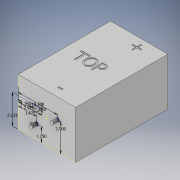
# Autodesk Inventor part: 12S Module
Saved by Autodesk Inventor 2017 (Build 210142000, 142)
## iProperties
Created: 2021-02-12
Part Number: 12S Module
Material: Generic
Document SubType Name: Modeling
Designer: Win240
Density: 1 g/cm^3
Appearance: Default
Author: Win240
Autodesk Inventor part; units mm, degrees
ref_plane "YZ Plane" through (0, 0, 0) normal (1, 0, 0) x (0, 1, 0)
ref_plane "XZ Plane" through (0, 0, 0) normal (0, 1, 0) x (-1, 0, 0)
ref_plane "XY Plane" through (0, 0, 0) normal (0, 0, 1) x (1, 0, 0)
sketch "Sketch1" plane through (0, 0, 0) normal (0, 0, 1) x (1, 0, 0)
  line L0 (-65.0875, -53.975) -> (65.0875, -53.975)
  line L1 (65.0875, -53.975) -> (65.0875, 53.975)
  line L2 (65.0875, 53.975) -> (-65.0875, 53.975)
  line L3 (-65.0875, 53.975) -> (-65.0875, -53.975)
  line L4 (-65.0875, -53.975) -> (65.0875, 53.975) construction
  line L5 (65.0875, -53.975) -> (-65.0875, 53.975) construction
  point P0 (0, 0)
  dimension "d0" = 130.175
  dimension "d1" = 107.95
  constraints: 12 end point, 2 midpoint, 2 parallel, 1 horizontal, 1 perpendicular
  measures "d0" distance of L0.start L0.end
  measures "d1" distance of L0.end L1.end
extrude "Extrusion1" add sketch "Sketch1" along normal blind 209.55
sketch "Sketch2" plane through (0, 0, 209.55) normal (0, 0, 1) x (1, 0, 0)
  line L0 (-65.0875, -53.975) -> (65.0875, -53.975) construction
  line L1 (-65.0875, 53.975) -> (-65.0875, -53.975) construction
  circle A0 centre (-23.8125, -22.225) radius 4
  circle A1 centre (23.8125, 9.525) radius 4
  line L2 (-11.1125, 12.065) -> (-33.3375, 12.065)
  line L3 (-33.3375, 12.065) -> (-33.3375, 13.335)
  line L4 (-33.3375, 13.335) -> (-11.1125, 13.335)
  line L5 (-11.1125, 13.335) -> (-11.1125, 12.065)
  line L6 (-33.3375, 12.7) -> (-65.0875, 12.7) construction
  point P0 (0, 0)
  dimension "d4" = 31.75
  dimension "d5" = 41.275
  dimension "d6" = 8
  dimension "d7" = 63.5
  dimension "d8" = 88.9
  dimension "d13" = 31.75
  dimension "d14" = 53.975
  dimension "d15" = 66.675
  dimension "d16" = 1.27
  constraints: 10 end point, 2 centre point, 2 horizontal, 2 parallel, 1 equal radius, 1 midpoint, 1 perpendicular, 1 point on line
  measures "d4" distance from line of A0.centre L0
  measures "d5" distance from line of A0.centre L1
  measures "d6" diameter of A0
  measures "d7" distance from line of A1.centre L0
  measures "d8" distance from line of A1.centre L1
  measures "d13" distance between parallel lines of L3 L1
  measures "d14" distance between parallel lines of L5 L1
  measures "d15" distance between parallel lines of L0 L6
  measures "d16" distance of L4.end L2.start
extrude "Extrusion2" add sketch "Sketch2" along normal blind 12.7
sketch "Sketch3" plane through (0, 0, 0) normal (0, 0, -1) x (-1, 0, 0)
  circle A0 centre (-23.8125, 9.525) radius 4 projected
  circle A1 centre (23.8125, -22.225) radius 4 projected
  line L0 (33.3375, 12.065) -> (11.1125, 12.065) projected
  line L1 (11.1125, 12.065) -> (11.1125, 13.335) projected
  line L2 (11.1125, 13.335) -> (33.3375, 13.335) projected
  line L3 (33.3375, 13.335) -> (33.3375, 12.065) projected
  point P0 (0, 0)
extrude "Extrusion3" add sketch "Sketch3" along normal blind 12.7
sketch "Sketch4" plane through (-33.3375, 13.335, 0) normal (0, 1, 0) x (1, 0, 0)
  line L0 (0, 12.7) -> (22.225, 12.7) projected
  line L1 (22.225, 0) -> (22.225, 12.7) projected
  line L2 (0, 0) -> (0, 12.7) projected
  line L3 (22.225, -209.55) -> (22.225, -222.25) projected
  line L4 (22.225, -222.25) -> (0, -222.25) projected
  line L5 (0, -209.55) -> (0, -222.25) projected
  line L6 (16.51, -219.71) -> (5.715, -219.71)
  line L7 (5.715, -219.71) -> (5.715, -215.265)
  line L8 (5.715, -215.265) -> (16.51, -215.265)
  line L9 (16.51, -215.265) -> (16.51, -219.71)
  line L10 (16.51, 5.715) -> (5.715, 5.715)
  line L11 (5.715, 5.715) -> (5.715, 10.16)
  line L12 (5.715, 10.16) -> (16.51, 10.16)
  line L13 (16.51, 10.16) -> (16.51, 5.715)
  line L14 (5.715, 10.16) -> (0, 12.7) construction
  line L15 (16.51, 10.16) -> (22.225, 12.7) construction
  line L16 (22.225, -222.25) -> (16.51, -219.71) construction
  line L17 (5.715, -219.71) -> (0, -222.25) construction
  point P0 (33.3375, 0)
  dimension "d17" = 10.795
  dimension "d18" = 6.985
  dimension "d19" = 2.54
  constraints: 24 end point, 5 equal length, 4 parallel, 2 horizontal, 2 perpendicular
  measures "d17" distance of L11.end L12.end
  measures "d18" distance between parallel lines of L10 L0
  measures "d19" distance between parallel lines of L12 L0
extrude "Extrusion4" cut sketch "Sketch4" against normal up to surface (1.27 mm away)
fillet "Fillet1" radius 3.175 4 edges at (-33.3375, 12.7, -12.7) (-11.1125, 12.7, -12.7) (-33.3375, 12.7, 222.25) (-11.1125, 12.7, 222.25)
thread "Thread1" size "M8x1.25" class "6g" standard "ANSI Metric M Profile" full length
thread "Thread2" size "M8x1.25" class "6g" standard "ANSI Metric M Profile" full length
thread "Thread3" size "M8x1.25" class "6g" standard "ANSI Metric M Profile" full length
thread "Thread4" size "M8x1.25" class "6g" standard "ANSI Metric M Profile" full length
sketch "Sketch5" plane through (-65.0875, 53.975, 0) normal (0, 1, 0) x (1, 0, 0)
  line L0 (25.2364, -11.8087) -> (114.825, -11.8087) construction
  line L1 (114.825, -11.8087) -> (114.825, -199.7093) construction
  line L2 (114.825, -199.7093) -> (25.2364, -199.7093) construction
  line L3 (25.2364, -199.7093) -> (25.2364, -11.8087) construction
  line L4 (91.6181, -23.1502) -> (83.0142, -23.1502)
  line L5 (83.0142, -23.1502) -> (83.0142, -31.7541)
  line L6 (83.0142, -31.7541) -> (80.1737, -31.7541)
  line L7 (80.1737, -31.7541) -> (80.1737, -23.1502)
  line L8 (80.1737, -23.1502) -> (71.5698, -23.1502)
  line L9 (71.5698, -23.1502) -> (71.5698, -20.4126)
  line L10 (71.5698, -20.4126) -> (80.1737, -20.4126)
  line L11 (80.1737, -20.4126) -> (80.1737, -11.8087)
  line L12 (80.1737, -11.8087) -> (83.0142, -11.8087)
  line L13 (83.0142, -11.8087) -> (83.0142, -20.4126)
  line L14 (83.0142, -20.4126) -> (91.6181, -20.4126)
  line L15 (91.6181, -20.4126) -> (91.6181, -23.1502)
  line L16 (33.7374, -116.5476) -> (33.7374, -94.1528)
  line L17 (33.7374, -94.1528) -> (25.2158, -94.1528)
  line L18 (25.2158, -94.1528) -> (25.2158, -91.1476)
  line L19 (25.2158, -91.1476) -> (45.6346, -91.1476)
  line L20 (45.6346, -91.1476) -> (45.6346, -94.1528)
  line L21 (45.6346, -94.1528) -> (37.1131, -94.1528)
  line L22 (37.1131, -94.1528) -> (37.1131, -116.5476)
  line L23 (37.1131, -116.5476) -> (33.7374, -116.5476)
  spline S0 degree 2 poles (66.1769, -94.0499) (67.6178, -95.7377) (69.2233, -100.6778) (69.2233, -103.8476) knots 0 0 0 1 2 2 2
  spline S1 degree 2 poles (69.2233, -103.8476) (69.2233, -106.9351) (67.6589, -111.9369) (66.1769, -113.6248) knots 0 0 0 1 2 2 2
  spline S2 degree 2 poles (66.1769, -113.6248) (64.6126, -115.3949) (60.4753, -117.0828) (57.9847, -117.0828) knots 0 0 0 1 2 2 2
  spline S3 degree 2 poles (57.9847, -117.0828) (55.4118, -117.0828) (51.2951, -115.3332) (49.7925, -113.6248) knots 0 0 0 1 2 2 2
  spline S4 degree 2 poles (49.7925, -113.6248) (48.3311, -111.9369) (46.7667, -106.9763) (46.7667, -103.8476) knots 0 0 0 1 2 2 2
  spline S5 degree 2 poles (46.7667, -103.8476) (46.7667, -100.6572) (48.3516, -95.7995) (49.8131, -94.0499) knots 0 0 0 1 2 2 2
  spline S6 degree 2 poles (49.8131, -94.0499) (51.2951, -92.362) (55.4324, -90.6125) (57.9847, -90.6125) knots 0 0 0 1 2 2 2
  spline S7 degree 2 poles (57.9847, -90.6125) (60.5782, -90.6125) (64.7361, -92.4238) (66.1769, -94.0499) knots 0 0 0 1 2 2 2
  spline S8 degree 2 poles (65.7035, -103.8476) (65.7035, -101.3364) (64.6126, -97.4462) (63.6246, -96.17) knots 0 0 0 1 2 2 2
  spline S9 degree 2 poles (63.6246, -96.17) (62.616, -94.8526) (59.7755, -93.5353) (58.0053, -93.5353) knots 0 0 0 1 2 2 2
  spline S10 degree 2 poles (58.0053, -93.5353) (56.1734, -93.5353) (53.4152, -94.8115) (52.3654, -96.17) knots 0 0 0 1 2 2 2
  spline S11 degree 2 poles (52.3654, -96.17) (51.3568, -97.4667) (50.2865, -101.3776) (50.2865, -103.8476) knots 0 0 0 1 2 2 2
  spline S12 degree 2 poles (50.2865, -103.8476) (50.2865, -108.8494) (54.4855, -114.1599) (58.0053, -114.1599) knots 0 0 0 1 2 2 2
  spline S13 degree 2 poles (58.0053, -114.1599) (61.5251, -114.1599) (65.7035, -108.8494) (65.7035, -103.8476) knots 0 0 0 1 2 2 2
  spline S14 degree 2 poles (88.9834, -98.8047) (88.9834, -100.4514) (87.8102, -103.4154) (86.7604, -104.4445) knots 0 0 0 1 2 2 2
  spline S15 degree 2 poles (86.7604, -104.4445) (85.4431, -105.7413) (81.8821, -107.0792) (79.1651, -107.0792) knots 0 0 0 1 2 2 2
  line L24 (79.1651, -107.0792) -> (76.304, -107.0792)
  line L25 (76.304, -107.0792) -> (76.304, -116.5476)
  line L26 (76.304, -116.5476) -> (72.9283, -116.5476)
  line L27 (72.9283, -116.5476) -> (72.9283, -91.1476)
  line L28 (72.9283, -91.1476) -> (79.3092, -91.1476)
  spline S16 degree 2 poles (79.3092, -91.1476) (81.5734, -91.1476) (84.7432, -91.8886) (85.9576, -92.7326) knots 0 0 0 1 2 2 2
  spline S17 degree 2 poles (85.9576, -92.7326) (87.3779, -93.7) (88.9834, -96.6846) (88.9834, -98.8047) knots 0 0 0 1 2 2 2
  spline S18 degree 2 poles (85.4636, -98.9076) (85.4636, -97.5902) (84.558, -95.6554) (83.6317, -95.0379) knots 0 0 0 1 2 2 2
  spline S19 degree 2 poles (83.6317, -95.0379) (82.829, -94.5027) (80.6883, -94.0705) (79.1034, -94.0705) knots 0 0 0 1 2 2 2
  line L29 (79.1034, -94.0705) -> (76.304, -94.0705)
  line L30 (76.304, -94.0705) -> (76.304, -104.1975)
  line L31 (76.304, -104.1975) -> (78.6093, -104.1975)
  spline S20 degree 2 poles (78.6093, -104.1975) (80.6677, -104.1975) (83.1995, -103.5389) (84.0228, -102.6744) knots 0 0 0 1 2 2 2
  spline S21 degree 2 poles (84.0228, -102.6744) (84.7844, -101.9128) (85.4636, -100.122) (85.4636, -98.9076) knots 0 0 0 1 2 2 2
  line L32 (80.0296, -190.6172) -> (70.4171, -190.6172)
  line L33 (70.4171, -190.6172) -> (70.4171, -187.5297)
  line L34 (70.4171, -187.5297) -> (80.0296, -187.5297)
  line L35 (80.0296, -187.5297) -> (80.0296, -190.6172)
  point P0 (65.0875, 0)
  constraints: 2 other
extrude "Extrusion7" cut sketch "Sketch5" against normal blind 0.762
sketch "Sketch6" plane through (0, 0, 0) normal (0, 0, -1) x (-1, 0, 0)
  circle A0 centre (8.3375, 46.3906) radius 3.175
  point P0 (0, 0)
  dimension "d31" = 6.35
  constraints: 1 centre point
  measures "d31" diameter of A0
sketch "Sketch7" plane through (-8.3375, 46.3906, -58.42) normal (0, 0, -1) x (-1, 0, 0)
  circle A0 centre (0, 0) radius 3.175 projected
  line L0 (-16.51, -7.3025) -> (16.51, -7.3025)
  line L1 (16.51, -7.3025) -> (16.51, 7.3025)
  line L2 (16.51, 7.3025) -> (-16.51, 7.3025)
  line L3 (-16.51, 7.3025) -> (-16.51, -7.3025)
  line L4 (-16.51, -7.3025) -> (16.51, 7.3025) construction
  line L5 (16.51, -7.3025) -> (-16.51, 7.3025) construction
  point P0 (-8.3375, -46.3906)
  dimension "d34" = 14.605
  dimension "d35" = 33.02
  constraints: 12 end point, 2 midpoint, 2 parallel, 1 horizontal, 1 perpendicular
  measures "d34" distance of L2.end L0.start
  measures "d35" distance of L1.end L2.end
body "Solid1"
